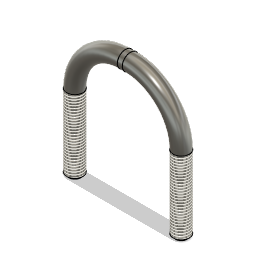
0.883.0500 - Etrier de 10x61x70 - IGTE 21400_17 Rep. 75 (Autodesk Fusion 360 design; units mm, degrees)
Autodesk Fusion 360 part; units mm, degrees
note: some values were not read from the file. Chosen so that the rebuilt part matches the saved one: which face or edge a step refers to; how an offset face is resized.
sketch "Sketch3" plane through (0, 0, 0) normal (0, 0, 1) x (1, 0, 0)
  line L0 (0, 0) -> (32, 0) construction
  line L1 (0, 0) -> (0, 48) construction
  line L2 (0, 0) -> (-32, 0) construction
  line L3 (32, 0) -> (32, -45)
  line L4 (-32, 0) -> (-32, -45)
  circle A0 centre (0, 0) radius 24.5 construction
  circle A1 centre (0, 0) radius 30.5 construction
  line L5 (0, 30.5) -> (-1.5, 30.5)
  line L6 (-32, 0) -> (-32, 0)
  arc A2 (-1.5, 30.5) -> (-32, 0) centre (-1.5, 0) ccw
  line L7 (32, 0) -> (32, 0)
  arc A3 (32, 0) -> (1.5, 30.5) centre (1.5, 0) ccw
  line L8 (0, 30.5) -> (1.5, 30.5)
  dimension "d22" = 32
  dimension "d23" = 45
  dimension "d24" = 45
  dimension "d25" = 49
  dimension "d26" = 6
  dimension "d27" = 30.5
  constraint coincident L0.start L1.start
  constraint perpendicular L0 L1
  constraint symmetric L0.start L1 L2.start
  constraint symmetric L0.end L1 L2.end
  constraint vertical L3
  constraint vertical L4
  constraint horizontal L0
  constraint coincident A1 L5.start
  constraint coincident L1 L5.start
  constraint tangent A1 L5
  constraint perpendicular L1 L5
  constraint tangent L5 A2
  constraint symmetric L1 L2.end L0.end
  constraint symmetric L1 L5.end A3.end
  constraint symmetric L1 A2 A3
  measures "d22" distance of L0.start L0.end
  measures "d23" distance of L0.end L3.end
  measures "d24" distance of L2.end L4.end
  measures "d25" diameter of A0
  measures "d27" radius of A2
sketch "Sketch4" plane through (0, 0, 0) normal (1, 0, 0) x (0, 0, -1)
  circle A0 centre (0, 30.5) radius 5
  point P0 (0, 30.5)
  dimension "d28" = 10
  constraint coincident P0 A0.centre
  measures "d28" diameter of A0
sweep "Sweep2" add profiles "Sketch4" path "Sketch3" along L3 A3 L8 L5 A2 L4 section 1
chamfer "Chamfer2" distance 1.5 angle 45 2 edges at (-33.8081, -45, 4.6616) (30.1919, -45, 4.6616)
thread "Thread3" "ISO Metric profile 10.0 M10x1.5 6g" major diameter 9.85 minor diameter 8.141 pitch 1.5 angle 60 resizes the face on face at (-31.5022, -14.5, -4.9752)
thread "Thread4" "ISO Metric profile 10.0 M10x1.5 6g"
equation "d22 = ( 64 / 2 ) * 1 mm"
